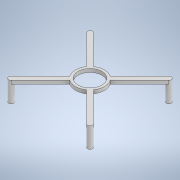
# Autodesk Inventor part: expo6
Saved by Autodesk Inventor 2020 (Build 240168000, 168)
## iProperties
Created: 2020-02-19
Part Number: expo6
Material: Generic
Document SubType Name: Modeling
Designer: Aryan
Density: 1 g/cm^3
Appearance: Default
Author: Aryan
Autodesk Inventor part; units mm, degrees
ref_plane "YZ Plane" through (0, 0, 0) normal (1, 0, 0) x (0, 1, 0)
ref_plane "XZ Plane" through (0, 0, 0) normal (0, 1, 0) x (-1, 0, 0)
ref_plane "XY Plane" through (0, 0, 0) normal (0, 0, 1) x (1, 0, 0)
sketch "Sketch1" plane through (0, 0, 0) normal (0, 1, 0) x (-1, 0, 0)
  line L0 (0, 0) -> (23.1577, -23.1577)
  line L1 (0, 0) -> (32.75, 0) construction
  circle A0 centre (23.1577, -23.1577) radius 1.5
  dimension "d0" = 32.75
  dimension "d1" = 45
  dimension "d2" = 3
  constraints: 4 end point, 1 centre point, 1 coincident, 1 equal length, 1 horizontal
  measures "d0" distance of L0.start L0.end
  measures "d1" angle of L0 L1
  measures "d2" diameter of A0
extrude "Extrusion1" add sketch "Sketch1" along normal blind 10
sketch "Sketch2" plane through (-23.1577, 0, -23.1577) normal (0, -1, 0) x (1, 0, 0)
  line L0 (23.1577, 23.1577) -> (46.3155, 46.3155)
  line L1 (23.1577, 23.1577) -> (55.9077, 23.1577) construction
  circle A0 centre (46.3155, 46.3155) radius 1.5
  dimension "d5" = 32.75
  dimension "d6" = 45
  dimension "d7" = 3
  constraints: 4 end point, 1 centre point, 1 coincident, 1 equal length, 1 horizontal
  measures "d5" distance of L0.start L0.end
  measures "d6" angle of L1 L0
  measures "d7" diameter of A0
extrude "Extrusion2" add sketch "Sketch2" against normal blind 10
sketch "Sketch3" plane through (-23.1577, 0, -23.1577) normal (0, -1, 0) x (1, 0, 0)
  line L0 (23.1577, 23.1577) -> (0, 46.3155)
  line L1 (23.1577, 23.1577) -> (55.9077, 23.1577) construction
  circle A0 centre (0, 46.3155) radius 1.5
  dimension "d10" = 32.75
  dimension "d11" = 135
  dimension "d12" = 3
  constraints: 4 end point, 1 centre point, 1 coincident, 1 equal length, 1 horizontal
  measures "d10" distance of L0.start L0.end
  measures "d11" angle of L1 L0
  measures "d12" diameter of A0
extrude "Extrusion3" add sketch "Sketch3" against normal blind 10
sketch "Sketch4" plane through (-23.1577, 10, -23.1577) normal (0, 1, 0) x (1, 0, 0)
  line L0 (23.1577, -23.1577) -> (46.3155, 0)
  line L1 (23.1577, -23.1577) -> (55.9077, -23.1577) construction
  circle A0 centre (46.3155, 0) radius 1.5
  dimension "d15" = 32.75
  dimension "d16" = 45
  dimension "d17" = 3
  constraints: 4 end point, 1 centre point, 1 coincident, 1 equal length, 1 horizontal
  measures "d15" distance of L0.start L0.end
  measures "d16" angle of L1 L0
  measures "d17" diameter of A0
extrude "Extrusion4" add sketch "Sketch4" against normal blind 10
sketch "Sketch5" plane through (23.1577, 10, -23.1577) normal (0, 1, 0) x (1, 0, 0)
  circle A0 centre (0, 0) radius 1.5 projected
  circle A1 centre (-46.3155, -46.3155) radius 1.5 projected
  line L0 (0, 0) -> (-46.3155, -46.3155) construction
  line L1 (-1.0607, 1.0607) -> (-47.3762, -45.2548)
  line L2 (-45.2548, -47.3762) -> (1.0607, -1.0607)
  arc A2 (1.0607, -1.0607) -> (-1.0607, 1.0607) centre (0, 0) ccw
  arc A3 (-47.3762, -45.2548) -> (-45.2548, -47.3762) centre (-46.3155, -46.3155) ccw
  point P0 (-23.1577, -23.1577)
  point P1 (-23.1577, -23.1577)
  dimension "d20" = 3
  constraints: 8 end point, 4 point on circle, 4 tangent, 2 centre point, 1 midpoint, 1 parallel
  measures "d20" diameter of A3
extrude "Extrusion5" add sketch "Sketch5" along normal blind 2
sketch "Sketch6" plane through (-23.1577, 10, -23.1577) normal (0, 1, 0) x (1, 0, 0)
  circle A0 centre (46.3155, -46.3155) radius 1.5 projected
  line L0 (46.3155, -46.3155) -> (0, 0) construction
  line L1 (47.3762, -45.2548) -> (1.0607, 1.0607)
  line L2 (-1.0607, -1.0607) -> (45.2548, -47.3762)
  arc A1 (45.2548, -47.3762) -> (47.3762, -45.2548) centre (46.3155, -46.3155) ccw
  arc A2 (1.0607, 1.0607) -> (-1.0607, -1.0607) centre (0, 0) ccw
  point P0 (23.1577, -23.1577)
  point P1 (23.1577, -23.1577)
  dimension "d23" = 3
  constraints: 8 end point, 4 point on circle, 4 tangent, 2 centre point, 1 midpoint, 1 parallel
  measures "d23" diameter of A2
extrude "Extrusion6" add sketch "Sketch6" along normal blind 2
sketch "Sketch7" plane through (23.1577, 12, -23.1577) normal (0, 1, 0) x (1, 0, 0)
  circle A0 centre (-23.1577, -23.1577) radius 8.5
  dimension "d26" = 17
  constraints: 1 centre point, 1 coincident
  measures "d26" diameter of A0
extrude "Extrusion7" add sketch "Sketch7" against normal blind 2
sketch "Sketch8" plane through (23.1577, 12, -23.1577) normal (0, 1, 0) x (1, 0, 0)
  circle A0 centre (-23.1577, -23.1577) radius 7
  dimension "d29" = 14
  constraints: 1 centre point, 1 coincident
  measures "d29" diameter of A0
extrude "Extrusion8" cut sketch "Sketch8" against normal blind 2
body "Solid1"
